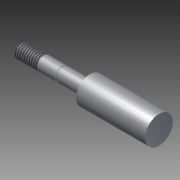
# Autodesk Inventor part: 13_1087_035
Saved by Autodesk Inventor 2014 (Build 180170000, 170)
## iProperties
Created: 2013-09-19
Part Number: 13_1087_035
Material: Allgemein
Document SubType Name: Modeling
Designer: vogel
Density: 1 g/cm^3
Appearance: Vorgabe
Author: vogel
Autodesk Inventor part; units mm, degrees
ref_plane "YZ Plane" through (0, 0, 0) normal (1, 0, 0) x (0, 1, 0)
ref_plane "XZ Plane" through (0, 0, 0) normal (0, 1, 0) x (-1, 0, 0)
ref_plane "XY Plane" through (0, 0, 0) normal (0, 0, 1) x (1, 0, 0)
sketch "Skizze1" plane through (0, 0, 0) normal (0, 0, 1) x (1, 0, 0)
  line L0 (-8, 0) -> (48, 0) projected
  line L1 (0, -0.6) -> (0, 3.6) projected
  line L2 (0, 1.5) -> (9, 1.5)
  line L3 (9, 1.15) -> (9.64, 1.15)
  line L4 (9.64, 1.15) -> (9.64, 1.5)
  line L5 (9.64, 1.5) -> (15, 1.5)
  line L6 (15, 1.5) -> (15, 3)
  line L7 (15, 3) -> (40, 3)
  line L8 (40, 3) -> (40, 0)
  line L9 (40, 0) -> (0, 0)
  line L10 (0, 0) -> (0, 1.5)
  line L11 (9, 1.5) -> (9, 1.15)
  dimension "d0" = 3
  dimension "d1" = 2.3
  dimension "d2" = 9
  dimension "d3" = 0.64
  dimension "d4" = 3
  dimension "d5" = 15
  dimension "d6" = 40
  dimension "d7" = 6
  constraints: 20 end point, 5 perpendicular, 3 parallel, 2 collinear, 1 midpoint, 1 point on line
  measures "d0" diameter of L2 L0
  measures "d1" diameter of L3 L0
  measures "d2" distance of L2.start L2.end
  measures "d3" distance of L3.start L3.end
  measures "d4" diameter of L5 L0
  measures "d5" distance between parallel lines of L6 L1
  measures "d6" distance between parallel lines of L8 L1
  measures "d7" diameter of L7 L0
revolve "Umdrehung1" add sketch "Skizze1" angle 360 about axis through (-10, 0, 0) along (1, 0, 0)
thread "Gewinde2" size "M3x0.5" class "6g" standard "ANSI Metric M Profile" length 7
chamfer "Fase1" distance 1 angle 45 2 edges at (15, -3, 0) (40, -3, 0)
